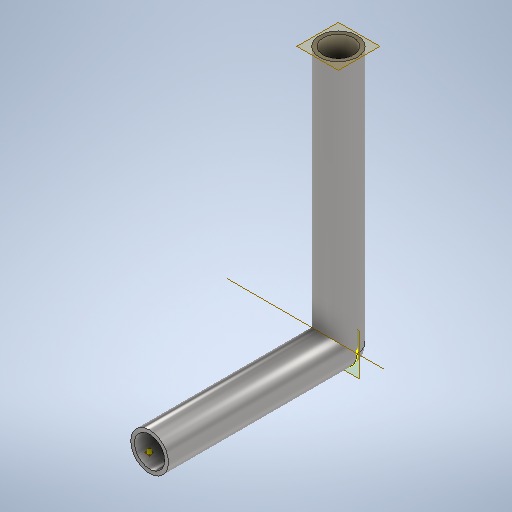
# Autodesk Inventor part: Z3
Saved by Autodesk Inventor 2025.2 (Build 292293000, 293)
## iProperties
Created: 2025-03-23
Part Number: Z3
Material: Steel, Alloy
Document SubType Name: Modeling
Designer: MSIGAMING
Mass: 8742.42 g
Surface Area: 2318.5 cm^2
Volume: 1130.97 cm^3
Density: 7.73 g/cm^3
Appearance: Semi-Polished
Author: MSIGAMING
Autodesk Inventor part; units mm, degrees
ref_plane "YZ Plane" through (0, 0, 0) normal (1, 0, 0) x (0, 1, 0)
ref_plane "XY Plane" through (0, 0, 0) normal (0, 0, 1) x (1, 0, 0)
sketch "Sketch1" plane through (0, 0, 0) normal (0, 0, 1) x (1, 0, 0)
  circle A0 centre (0, 0) radius 50
  circle A1 centre (0, 0) radius 40
  dimension "d0" = 100
  dimension "d1" = 80
  constraints: 2 centre point, 2 coincident
  measures "d0" diameter of A0
  measures "d1" diameter of A1
extrude "Extrusion1" add sketch "Sketch1" against normal blind 500
ref_plane "Work Plane1" through (0, 0, -500) normal (0, 0, -1) x (-1, 0, 0)
sketch "Sketch2" plane through (0, 0, -500) normal (0, 0, -1) x (-1, 0, 0)
  circle A0 centre (0, 0) radius 50 projected
  circle A1 centre (0, 0) radius 40 projected
  line L0 (0, 0) -> (0, 50)
  constraints: 2 end point, 1 vertical, 1 vertical alignment, 1 other
sketch "Sketch3" plane through (0, 0, 0) normal (0, 1, 0) x (-1, 0, 0)
  point P0 (0, 0)
sketch "Sketch4" plane through (0, 0, 0) normal (0, 1, 0) x (-1, 0, 0)
  line L0 (70, -500) -> (-70, -500) projected
  line L1 (-50, -500) -> (50, -500) projected
  circle A0 centre (0, -500) radius 40
  circle A1 centre (0, -500) radius 50
  point P0 (0, 0)
  point P1 (40, -500)
  point P2 (-40, -500)
  dimension "d5" = 80
  dimension "d6" = 100
  constraints: 2 centre point, 1 coincident, 1 midpoint
  measures "d5" diameter of A0
  measures "d6" diameter of A1
sketch "Sketch6" plane through (0, 0, 0) normal (0, 1, 0) x (-1, 0, 0)
  point P0 (0, 0)
sketch "Sketch7" plane through (0, 0, 0) normal (0, 1, 0) x (-1, 0, 0)
  line L0 (-40, -500) -> (-40, -500) projected
  circle A0 centre (0, -500) radius 40
  line L1 (-50, -500) -> (-50, -500) projected
  circle A1 centre (0, -500) radius 50
  point P0 (0, 0)
  point P1 (50, -400)
  point P2 (40, -400)
  constraints: 1 coincident, 1 point on line, 6 other
ref_plane "Work Plane4" through (50, 0, -500) normal (0, 0.7071, -0.7071) x (-1, 0, 0)
split "Split2" plane through (50, 0, -500) removes the side toward (0, 0.7071, -0.7071)
extrude "Extrusion3" add sketch "Sketch7" along normal blind 680
revolve "Revolution2" add sketch "Sketch4" angle 90 about axis through (0, 0, -500) along (-1, 0, 0) picked at (-46.3464, -503.2515) contours A1 L0 A0
ref_plane "Work Plane5" through (0, 680, -500) normal (0, 1, 0) x (1, 0, 0)
body "Solid1"
